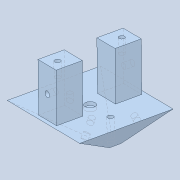
# Autodesk Inventor part: Part1
Saved by Autodesk Inventor 2020 (Build 240168000, 168)
## iProperties
Created: 2019-06-12
Part Number: Part1
Material: ABS Plastic
Document SubType Name: Modeling
Designer: kimhos
Density: 1.06 g/cm^3
Appearance: Light Steel Blue
Author: kimhos
Autodesk Inventor part; units mm, degrees
ref_plane "YZ Plane" through (0, 0, 0) normal (1, 0, 0) x (0, 1, 0)
ref_plane "XZ Plane" through (0, 0, 0) normal (0, 1, 0) x (-1, 0, 0)
sketch "Sketch1" plane through (0, 0, 0) normal (0, 1, 0) x (-1, 0, 0)
  line L0 (-8, 0) -> (-8, 8)
  line L1 (-8, 8) -> (8, 8)
  line L2 (8, 8) -> (8, -8)
  line L3 (8, -8) -> (-8, -8)
  line L4 (-8, -8) -> (-8, 0)
  circle A0 centre (0, 0) radius 1.5
  line L5 (8, 8) -> (8, 4.5)
  line L6 (8, 4.5) -> (5, 4.5)
  line L7 (-8, 8) -> (-8, 4.5)
  line L8 (-8, 4.5) -> (-5, 4.5)
  line L9 (0, 0) -> (0, 4.5)
  dimension "d0" = 8
  dimension "d1" = 8
  dimension "d2" = 16
  dimension "d3" = 16
  dimension "d4" = 16
  dimension "d5" = 8
  dimension "d25" = 3
  dimension "d95" = 3.5
  dimension "d96" = 3
  dimension "d106" = 3.5
  dimension "d107" = 3
  dimension "d196" = 4.5
  constraints: 20 end point, 4 perpendicular, 3 point on line, 1 centre point, 1 coincident, 1 vertical
  measures "d0" distance of point (0, 0) L0.start
  measures "d1" distance of L0.start L0.end
  measures "d2" distance of L0.end L1.end
  measures "d3" distance of L1.end L2.end
  measures "d4" distance of L2.end L3.end
  measures "d5" distance of L3.end L0.start
  measures "d25" diameter of A0
  measures "d95" distance of L1.end L5.end
  measures "d96" distance of L5.end L6.end
  measures "d106" distance of L0.end L7.end
  measures "d107" distance of L7.end L8.end
  measures "d196" distance of L9.start L9.end
ref_plane "Work Plane2" through (8, -4, 0) normal (0, -1, 0) x (0, 0, 1)
sketch "Sketch3" plane through (8, -4, 0) normal (0, -1, 0) x (0, 0, 1)
  line L0 (5.5, 8) -> (5.5, 7)
  line L1 (5.5, 7) -> (3.5, 7)
  line L2 (3.5, 7) -> (3.5, 9)
  line L3 (3.5, 9) -> (5.5, 9)
  line L4 (5.5, 9) -> (5.5, 8)
  line L5 (0, 8) -> (3.5, 8)
  dimension "d16" = 1
  dimension "d17" = 2
  dimension "d18" = 2
  dimension "d19" = 2
  dimension "d20" = 1
  dimension "d27" = 3.5
  constraints: 12 end point, 2 perpendicular, 1 midpoint, 1 point on line
  measures "d16" distance of L0.start L0.end
  measures "d17" distance of L0.end L1.end
  measures "d18" distance of L1.end L2.end
  measures "d19" distance of L2.end L3.end
  measures "d20" distance of L3.end L0.start
  measures "d27" distance of L5.start L5.end
loft "Loft1" add profiles "Sketch1", "Sketch3" contours L0 L1 L2 L3 L4 | A0 / all
sketch "Sketch5" plane through (-8, 0, -8) normal (0, 1, 0) x (1, 0, 0)
  line L0 (8, -8) -> (8, -12.5)
  circle A0 centre (8, -12.5) radius 0.5
  dimension "d28" = 4.5
  dimension "d29" = 1
  constraints: 2 end point, 1 centre point, 1 coincident, 1 vertical
  measures "d28" distance of L0.start L0.end
  measures "d29" diameter of A0
hole "Hole1" at (0, 0, 4.5) direction (0, -1, 0) diameter 1 depth 4
sketch "Sketch6" plane through (-8, 0, -8) normal (0, 1, 0) x (1, 0, 0)
  line L0 (8, -8) -> (10.8, -8)
  line L1 (16, 0) -> (16, -16) projected
  line L2 (10.8, -8) -> (10.8, -6)
  line L3 (10.8, -6) -> (15.3, -6)
  line L4 (15.3, -6) -> (15.3, -10)
  line L5 (15.3, -10) -> (10.8, -10)
  line L6 (10.8, -10) -> (10.8, -8)
  line L7 (15.3, -8) -> (16, -8)
  dimension "d180" = 2
  dimension "d181" = 4.5
  dimension "d182" = 4
  dimension "d183" = 4.5
  dimension "d184" = 2
  dimension "d185" = 0.7
  dimension "d197" = 2.8
  constraints: 14 end point, 3 perpendicular, 2 midpoint, 1 horizontal, 1 point on line, 1 vertical
  measures "d180" distance of L0.end L2.end
  measures "d181" distance of L2.end L3.end
  measures "d182" distance of L3.end L4.end
  measures "d183" distance of L4.end L5.end
  measures "d184" distance of L5.end L0.end
  measures "d185" distance of L7.start L7.end
  measures "d197" distance of L0.start L0.end
extrude "Extrusion1" add sketch "Sketch6" along normal blind 8.5
sketch "Sketch7" plane through (-8, 8.5, -8) normal (0, 1, 0) x (1, 0, 0)
  line L0 (8, -8) -> (13.5, -8)
  circle A0 centre (13.5, -8) radius 0.5
  circle A1 centre (13.5, -8) radius 0.75
  dimension "d48" = 5.5
  dimension "d49" = 1
  dimension "d57" = 1.5
  constraints: 2 centre point, 2 coincident, 2 end point, 1 horizontal
  measures "d48" distance of L0.start L0.end
  measures "d49" diameter of A0
  measures "d57" diameter of A1
hole "Hole2" at (5.5, 8.5, 0) direction (0, -1, 0) diameter 1 depth 2.5
sketch "Sketch8" plane through (-8, 0, -8) normal (0, 1, 0) x (1, 0, 0)
  line L0 (8, -8) -> (5.2, -8)
  line L1 (5.2, -8) -> (5.2, -6)
  line L2 (5.2, -6) -> (0.7, -6)
  line L3 (0.7, -6) -> (0.7, -10)
  line L4 (0.7, -10) -> (5.2, -10)
  line L5 (5.2, -10) -> (5.2, -8)
  line L6 (0.7, -8) -> (0, -8)
  dimension "d58" = 2.8
  dimension "d59" = 2
  dimension "d60" = 4.5
  dimension "d61" = 4
  dimension "d62" = 4.5
  dimension "d63" = 2
  dimension "d179" = 0.7
  constraints: 14 end point, 3 perpendicular, 2 horizontal, 1 midpoint, 1 point on line
  measures "d58" distance of L0.start L0.end
  measures "d59" distance of L0.end L1.end
  measures "d60" distance of L1.end L2.end
  measures "d61" distance of L2.end L3.end
  measures "d62" distance of L3.end L4.end
  measures "d63" distance of L4.end L0.end
  measures "d179" distance of L6.start L6.end
extrude "Extrusion2" add sketch "Sketch8" along normal blind 8.5
sketch "Sketch9" plane through (-8, 8.5, -8) normal (0, 1, 0) x (1, 0, 0)
  line L0 (8, -8) -> (2.5, -8)
  circle A0 centre (2.5, -8) radius 0.5
  circle A1 centre (2.5, -8) radius 0.75
  dimension "d66" = 5.5
  dimension "d67" = 1
  dimension "d75" = 1.5
  constraints: 2 centre point, 2 coincident, 2 end point, 1 horizontal
  measures "d66" distance of L0.start L0.end
  measures "d67" diameter of A0
  measures "d75" diameter of A1
hole "Hole3" at (-5.5, 8.5, 0) direction (0, -1, 0) diameter 1 depth 2.5
sketch "Sketch11" plane through (-7.3, 0, -2) normal (-1, 0, 0) x (0, 0, 1)
  line L0 (2, 0) -> (2, 4)
  circle A0 centre (2, 4) radius 0.5
  dimension "d85" = 4
  dimension "d86" = 1
  constraints: 2 end point, 1 centre point, 1 coincident, 1 vertical
  measures "d85" distance of L0.start L0.end
  measures "d86" diameter of A0
hole "Hole5" at (-7.3, 4, 0) direction (1, 0, 0) diameter 1 depth 1.5
sketch "Sketch13" plane through (-8, 0, -8) normal (-0.4961389, -0.8682431, 0) x (0.8682431, -0.4961389, 0)
  line L0 (0, 16) -> (0, 0) projected
  line L1 (0, 16) -> (0, 12.5)
  line L2 (0, 12.5) -> (4, 12.5)
  circle A0 centre (4, 12.5) radius 0.25
  point P0 (6.9459, 8)
  dimension "d97" = 3.5
  dimension "d98" = 0.5
  dimension "d118" = 4
  constraints: 4 end point, 1 centre point, 1 coincident, 1 perpendicular, 1 point on line
  measures "d97" distance of L0.start L1.end
  measures "d98" diameter of A0
  measures "d118" distance of L1.end L2.end
hole "Hole6" at (-4.527, -1.9846, 4.5) direction (0.4961389, 0.8682431, 0) diameter 1 depth 1
sketch "Sketch14" plane through (8, 0, -8) normal (0.4961389, -0.8682431, 0) x (0.8682431, 0.4961389, 0)
  line L0 (0, 16) -> (-8.0623, 13.5) projected
  line L1 (0, 16) -> (0, 12.5)
  line L2 (0, 0) -> (0, 16) projected
  line L3 (0, 12.5) -> (-4, 12.5)
  circle A0 centre (-4, 12.5) radius 0.25
  point P0 (-6.9459, 8)
  dimension "d108" = 3.5
  dimension "d109" = 0.5
  dimension "d117" = 4
  constraints: 4 end point, 1 centre point, 1 coincident, 1 perpendicular, 1 point on line
  measures "d108" distance of L0.start L1.end
  measures "d109" diameter of A0
  measures "d117" distance of L1.end L3.end
hole "Hole7" at (4.527, -1.9846, 4.5) direction (-0.4961389, 0.8682431, 0) diameter 1 depth 1
sketch "Sketch15" plane through (-8, 0, -8) normal (0, -0.9444968, -0.3285206) x (1, 0, 0)
  line L0 (0, 0) -> (16, 0) projected
  line L1 (0, 0) -> (8, 0)
  line L2 (8, 0) -> (8, 8.4687)
  circle A0 centre (8, 8.4687) radius 0.25
  dimension "d119" = 8
  dimension "d120" = 0.5
  constraints: 4 end point, 1 centre point, 1 coincident, 1 midpoint, 1 perpendicular
  measures "d119" distance of L0.start L1.end
  measures "d120" diameter of A0
hole "Hole8" at (0, -2.7821, -0.0014) direction (0, 0.9444968, 0.3285206) diameter 1 depth 1
sketch "Sketch17" plane through (-8, 0, -8) normal (0, 1, 0) x (1, 0, 0)
  line L0 (8, -8) -> (8, -3.5)
  circle A0 centre (8, -3.5) radius 0.25
  dimension "d128" = 4.5
  dimension "d129" = 0.5
  constraints: 2 end point, 1 centre point, 1 coincident, 1 vertical
  measures "d128" distance of L0.start L0.end
  measures "d129" diameter of A0
hole "Hole9" at (0, 0, -4.5) direction (0, -1, 0) diameter 1 depth 3
sketch "Sketch21" plane through (-8, 0, -8) normal (0, 1, 0) x (1, 0, 0)
  circle A0 centre (8, -8) radius 0.8
  dimension "d171" = 1.6
  constraints: 1 centre point, 1 coincident
  measures "d171" diameter of A0
hole "Hole12" at (0, 0, 0) direction (0, -1, 0) diameter 1.8 depth 0.6
sketch "Sketch22" plane through (7.3, 0, 2) normal (1, 0, 0) x (0, 0, -1)
  line L0 (2, 0) -> (2, 4)
  line L1 (2, 0) -> (6, 0) construction
  circle A0 centre (2, 4) radius 0.5
  dimension "d186" = 4
  dimension "d187" = 90
  dimension "d188" = 1
  constraints: 4 end point, 1 centre point, 1 coincident, 1 horizontal, 1 perpendicular, 1 vertical
  measures "d186" distance of L0.start L0.end
  measures "d187" angle of L1 L0
  measures "d188" diameter of A0
hole "Hole13" at (7.3, 4, 0) direction (-1, 0, 0) diameter 1 depth 1.5
sketch "Sketch23" plane through (-8, 0, -8) normal (0, 1, 0) x (1, 0, 0)
  line L0 (15.3, -10) -> (10.8, -10) projected
  line L1 (15.3, -10) -> (15.3, -15)
  point P0 (8, -8)
  dimension "d198" = 5
  constraints: 2 end point, 1 vertical
  measures "d198" distance of L0.start L1.end
ref_plane "Work Plane" through (8, 0, 0) normal (0, -1, 0) x (0, 0, 1)
body "Solid1"
